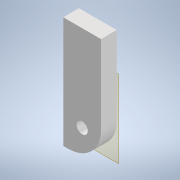
# Autodesk Inventor part: adapter
Saved by Autodesk Inventor 2020.1 (Build 241239000, 239)
## iProperties
Created: 2019-10-23
Part Number: adapter
Material: Generic
Document SubType Name: Modeling
Designer: jesse
Density: 1 g/cm^3
Appearance: Default
Author: jesse
Autodesk Inventor part; units mm, degrees
ref_plane "YZ Plane" through (0, 0, 0) normal (1, 0, 0) x (0, 1, 0)
ref_plane "XZ Plane" through (0, 0, 0) normal (0, 1, 0) x (-1, 0, 0)
ref_plane "XY Plane" through (0, 0, 0) normal (0, 0, 1) x (1, 0, 0)
ref_plane "Work Plane1" through (0, 0, 0) normal (0, 0, 1) x (1, 0, 0)
sketch "Sketch1" plane through (0, 0, 0) normal (0, 0, 1) x (1, 0, 0)
  line L0 (31.75, -13.716) -> (31.75, -6.096) projected
  arc A0 (25.146, -20.32) -> (31.75, -13.716) centre (25.146, -13.716) ccw projected
  line L1 (24.13, -20.32) -> (25.146, -20.32) projected
  circle A1 centre (27.94, -15.24) radius 1.1303 projected
  line L2 (31.75, -6.096) -> (31.75, -10.4198)
  line L3 (31.75, -10.4198) -> (24.13, -10.4198)
  line L4 (24.13, -10.4198) -> (24.13, -20.32)
  point P0 (0, 0)
  constraints: 6 end point, 1 perpendicular, 1 point on line, 1 vertical
extrude "Extrusion1" add sketch "Sketch1" along normal blind 3.175
body "Solid1"
